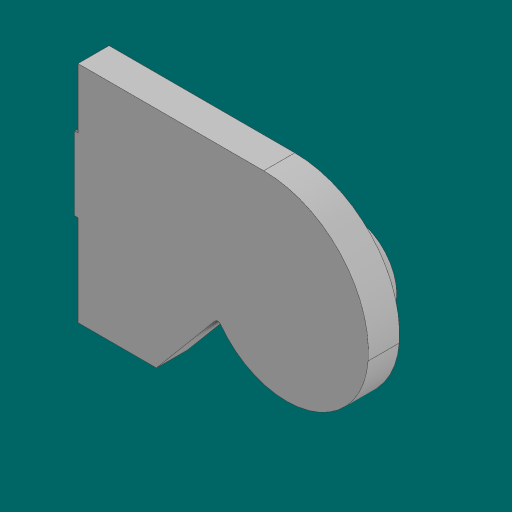
# Autodesk Inventor part: hs5_master
Saved by Autodesk Inventor 2024.3 (Build 283343000, 343)
## iProperties
Created: 2026-07-31
Part Number: hs5_master
Material: Generic
Document SubType Name: Modeling
Designer: penta
Density: 1 g/cm^3
Appearance: wall/default
OfanX: 36.000 mm
OfanY: 20.000 mm
OinletDiameter: 16.000 mm
wallThickness: 1.200 mm
OvoluteStartClearance: 0.500 mm
OvoluteStartY: 14.000 mm
Ovoulte1Dia: 13.000 mm
Ovoulte2Dia: 17.000 mm
OdiagOutletAngle: 50.00 deg
OfanZ: 4.000 mm
OinletChamfer: 1.000 mm
Author: penta
Autodesk Inventor part; units mm, degrees
ref_plane "YZ Plane" through (0, 0, 0) normal (1, 0, 0) x (0, 1, 0)
ref_plane "XZ Plane" through (0, 0, 0) normal (0, 1, 0) x (-1, 0, 0)
ref_plane "XY Plane" through (0, 0, 0) normal (0, 0, 1) x (1, 0, 0)
sketch "Sketch1" plane through (0, 0, 0) normal (0, 0, 1) x (1, 0, 0)
  line L0 (3, 35) -> (23, 35)
  line L1 (23, 35) -> (23, 15)
  line L2 (23, 15) -> (3, 15)
  line L3 (3, 15) -> (3, 35)
  line L4 (3, 15) -> (23, 35) construction
  circle A0 centre (36, 20) radius 8
  line L5 (0.6, 0) -> (0.6, 15.8)
  line L6 (1.2, 15.8) -> (0, 15.8)
  line L7 (0, 15.8) -> (0, 28.6)
  line L8 (0, 28.6) -> (1.2, 28.6)
  line L9 (0.6, 28.6) -> (0.6, 39)
  arc A1 (25.6077, 14) -> (49.8294, 19.525) centre (36.866, 20.5) ccw
  circle A2 centre (36, 20) radius 12 construction
  line L10 (0.6, 39) -> (32.8773, 39)
  line L11 (0.6, 0) -> (51, 0) construction
  circle A3 centre (5.3, 37.3) radius 1.4
  circle A4 centre (25.9, 17.1) radius 1.4
  arc A5 (3.3083, 35.6288) -> (7.2917, 35.6288) centre (5.3, 37.3) ccw
  line L12 (3.3083, 35.6288) -> (0.6, 38.8564)
  line L13 (7.2917, 35.6288) -> (9.1136, 37.8)
  line L14 (9.1136, 37.8) -> (32.8773, 37.8)
  line L15 (5.3, 37.3) -> (5.3, 39) construction
  arc A6 (49.8294, 19.525) -> (32.8773, 37.8) centre (32.8773, 20.8) ccw
  arc A7 (51.026, 19.435) -> (32.8773, 39) centre (32.8773, 20.8) ccw
  line L16 (25.6077, 14) -> (24.4077, 14)
  line L17 (24.4077, 14) -> (13.6672, 1.2)
  arc A8 (25.3867, 12.1415) -> (51.026, 19.435) centre (36.866, 20.5) ccw
  line L18 (13.6672, 1.2) -> (0.6, 1.2)
  line L19 (14.2268, 0) -> (24.442, 12.174)
  arc A9 (25.3867, 12.1415) -> (24.442, 12.174) centre (24.9016, 11.7883) ccw
  line L20 (1.2, 28.6) -> (1.2, 15.8)
  line L21 (14.2268, 0) -> (0.6, 0)
  circle A10 centre (36, 20) radius 11.7
  point P0 (13, 25)
  point P1 (0, 0)
  dimension "d28" = 24
  dimension "d0" = 20
  dimension "d2" = 16
  dimension "d8" = 10.4
  dimension "d9" = 15.8
  dimension "d10" = 12.8
  dimension "d18" = 13
  dimension "d20" = 36
  dimension "d22" = 25
  dimension "d23" = 2.8
  dimension "d24" = 20.6
  dimension "d25" = 20.2
  dimension "d26" = 12.9
  dimension "d27" = 7.9
  dimension "d29" = 20
  dimension "d30" = 1.2
  dimension "d31" = 50
  dimension "d32" = 1.2
  dimension "d33" = 51
  dimension "d34" = 1.2
  dimension "d36" = 14
  dimension "d37" = 1.2
  dimension "d39" = 1.2
  dimension "d40" = 0.6
  dimension "d41" = 13
  dimension "d42" = 17
  dimension "d43" = 50
  dimension "d55" = 23.4
  dimension "d66" = 1.2
  constraints: 44 end point, 12 point on circle, 10 centre point, 8 horizontal, 8 tangent, 6 point on line, 5 coincident, 5 vertical, 4 parallel, 3 midpoint, 2 perpendicular, 1 equal radius, 5 other
  measures "d0" distance of L1.end L2.end
  measures "d2" diameter of A0
  measures "d8" distance of L9.start L9.end
  measures "d9" distance of L5.end L5.start
  measures "d10" distance of L6.end L7.end
  measures "d18" horizontal distance of point (13, 25) point (0, 0)
  measures "d20" horizontal distance of A0.centre point (0, 0)
  measures "d22" vertical distance of point (0, 0) point (13, 25)
  measures "d23" diameter of A3
  measures "d24" horizontal distance of A4.centre A3.centre
  measures "d25" vertical distance of A4.centre A3.centre
  measures "d26" horizontal distance of A4.centre point (13, 25)
  measures "d27" vertical distance of point (13, 25) A4.centre
  measures "d29" vertical distance of point (0, 0) A0.centre
  measures "d30" radial gap between concentric circles of A5 A3
  measures "d31" angle of L10 L12
  measures "d32" distance between parallel lines of L14 L10
  measures "d33" distance of point (0, 0) L11.end
  measures "d34" distance of L16.start L16.end
  measures "d36" distance from line of point (0, 0) L16
  measures "d37" distance between parallel lines of L11 L18
  measures "d39" distance between parallel lines of L19 L17
  measures "d40" radius of A9
  measures "d41" radius of A1
  measures "d42" radius of A6
  measures "d43" angle of L11 L19
  measures "d55" diameter of A10
  measures "d66" distance of L6.start L6.end
sketch "Sketch2" plane through (0, 0, 0) normal (0, 0, 1) x (1, 0, 0)
  arc A0 (51.026, 19.435) -> (32.8773, 39) centre (32.8773, 20.8) ccw projected
  line L0 (0.6, 39) -> (32.8773, 39) projected
  arc A1 (25.3867, 12.1415) -> (51.026, 19.435) centre (36.866, 20.5) ccw projected
  arc A2 (25.3867, 12.1415) -> (24.442, 12.174) centre (24.9016, 11.7883) ccw projected
  line L1 (14.2268, 0) -> (24.442, 12.174) projected
  line L2 (0.6, 0) -> (0.6, 15.8) projected
  line L3 (1.2, 15.8) -> (0, 15.8) projected
  line L4 (0, 15.8) -> (0, 28.6) projected
  line L5 (0, 28.6) -> (1.2, 28.6) projected
  line L6 (0.6, 28.6) -> (0.6, 39) projected
  line L7 (14.2268, 0) -> (0.6, 0) projected
  point P0 (0, 0)
  point P1 (0.6, 15.8)
  constraints: 2 other
sketch "Sketch4" plane through (0, 0, 0) normal (0, 0, 1) x (1, 0, 0)
  line L0 (0.6, 39) -> (32.8773, 39) projected
  line L1 (3.3083, 35.6288) -> (0.6, 38.8564) projected
  arc A0 (3.3083, 35.6288) -> (7.2917, 35.6288) centre (5.3, 37.3) ccw projected
  line L2 (7.2917, 35.6288) -> (9.1136, 37.8) projected
  line L3 (9.1136, 37.8) -> (32.8773, 37.8) projected
  arc A1 (49.8294, 19.525) -> (32.8773, 37.8) centre (32.8773, 20.8) ccw projected
  arc A2 (51.026, 19.435) -> (32.8773, 39) centre (32.8773, 20.8) ccw projected
  arc A3 (25.6077, 14) -> (49.8294, 19.525) centre (36.866, 20.5) ccw projected
  arc A4 (25.3867, 12.1415) -> (51.026, 19.435) centre (36.866, 20.5) ccw projected
  line L4 (25.6077, 14) -> (24.4077, 14) projected
  arc A5 (25.3867, 12.1415) -> (24.442, 12.174) centre (24.9016, 11.7883) ccw projected
  line L5 (24.4077, 14) -> (13.6672, 1.2) projected
  line L6 (14.2268, 0) -> (24.442, 12.174) projected
  line L7 (14.2268, 0) -> (0.6, 0) projected
  line L8 (13.6672, 1.2) -> (0.6, 1.2) projected
  line L9 (1.2, 28.6) -> (1.2, 15.8) projected
  line L10 (0, 28.6) -> (1.2, 28.6) projected
  line L11 (0, 15.8) -> (0, 28.6) projected
  line L12 (1.2, 15.8) -> (0, 15.8) projected
  line L13 (0.6, 38.8564) -> (0.6, 39)
  line L14 (0.6, 1.2) -> (0.6, 0)
  point P0 (0, 0)
  constraints: 4 end point, 2 vertical
extrude "Extrusion3" add sketch "Sketch2" along normal blind 4 and the other way blind 1.4
extrude "Extrusion1" add sketch "Sketch2" against normal through all separate body
extrude "Extrusion2" add sketch "Sketch4" along normal through all bodies 2
sketch "Sketch5" plane through (0, 0, 0) normal (0, 0, 1) x (1, 0, 0)
  circle A0 centre (25.9, 17.1) radius 1.4 projected
  point P0 (0, 0)
extrude "Extrusion4" add sketch "Sketch5" along normal through all separate body
sketch "Sketch6" plane through (0, 0, 0) normal (0, 0, 1) x (1, 0, 0)
  circle A0 centre (36, 20) radius 11.7 projected
  point P0 (0, 0)
extrude "Extrusion5" add sketch "Sketch6" along normal through all bodies 3
sketch "Sketch7" plane through (0, 0, 0) normal (0, 0, 1) x (1, 0, 0)
  circle A0 centre (36, 20) radius 8 projected
  point P0 (0, 0)
extrude "Extrusion6" add sketch "Sketch7" against normal blind 8 bodies 3
chamfer "Chamfer2" distance 1 angle 45 1 edges at (28, 20, 0)
combine bodies "Combine3" operation type add bodies to combine 1 3 keep tools yes
combine bodies "Combine4" operation type subtract main body 2 bodies to subtract 3 keep tools yes
sketch "Sketch8" plane through (0, 0, 0) normal (0, 0, 1) x (1, 0, 0)
  circle A0 centre (36, 20) radius 11.7 projected
  point P0 (0, 0)
extrude "Extrusion7" add sketch "Sketch8" along normal through all separate body
split_face "Split1"
equation "\"d2\" = OinletDiameter"
equation "\"d20\" = OfanX"
equation "\"d29\" = OfanY"
equation "\"d30\" = wallThickness"
equation "\"d32\" = wallThickness"
equation "\"OfanX\" = 36"
equation "\"OfanY\" = 20"
equation "\"OinletDiameter\" = 16"
equation "\"wallThickness\" = 1.2"
equation "\"OvoluteStartClearance\" = 0.5"
equation "\"OvoluteStartY\" = 14"
equation "\"Ovoulte1Dia\" = 13"
equation "\"Ovoulte2Dia\" = 17"
equation "\"OdiagOutletAngle\" = 50deg"
equation "\"OfanZ\" = 4"
equation "\"OinletChamfer\" = 1"
